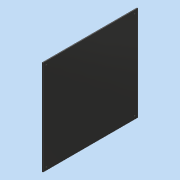
# Autodesk Inventor part: FrameBack
Saved by Autodesk Inventor 2016 (Build 200138000, 138)
## iProperties
Created: 2016-08-20
Part Number: FrameBack
Material: Dibond
Document SubType Name: Modeling
Designer: Sam
Density: 1 g/cm^3
Appearance: Generic
Author: Sam
Autodesk Inventor part; units mm, degrees
ref_plane "YZ Plane" through (0, 0, 0) normal (1, 0, 0) x (0, 1, 0)
ref_plane "XZ Plane" through (0, 0, 0) normal (0, 1, 0) x (-1, 0, 0)
ref_plane "XY Plane" through (0, 0, 0) normal (0, 0, 1) x (1, 0, 0)
sketch "Sketch1" plane through (0, 0, 0) normal (1, 0, 0) x (0, 1, 0)
  line L0 (0, 0) -> (360, 0)
  line L1 (360, 0) -> (360, -360)
  line L2 (360, -360) -> (0, -360)
  line L3 (0, -360) -> (0, 0)
  dimension "d0" = 360
  dimension "d1" = 360
  constraints: 8 end point, 2 parallel, 1 horizontal, 1 perpendicular
  measures "d0" distance of L1.end L2.end
  measures "d1" distance of L0.end L1.end
extrude "Extrusion1" add sketch "Sketch1" along normal blind 3
hole "Hole1" at (3, 12, -12) direction (-1, 0, 0) diameter 4 end through all
hole "Hole2" at (3, 12, -348) direction (-1, 0, 0) diameter 4 end through all
hole "Hole3" at (3, 348, -12) direction (-1, 0, 0) diameter 4 end through all
hole "Hole4" at (3, 348, -348) direction (-1, 0, 0) diameter 4 end through all
body "Solid1"
